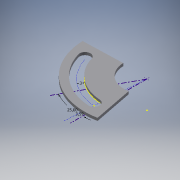
# Autodesk Inventor part: Fixação Painel
Saved by Autodesk Inventor 2019 (Build 230136000, 136)
## iProperties
Created: 2020-05-30
Part Number: Fixação Painel
Material: Generic
Document SubType Name: Modeling
Designer: luiza
Density: 1 g/cm^3
Appearance: Default
Author: luiza
Autodesk Inventor part; units mm, degrees
ref_plane "YZ Plane" through (0, 0, 0) normal (1, 0, 0) x (0, 1, 0)
ref_plane "XZ Plane" through (0, 0, 0) normal (0, 1, 0) x (-1, 0, 0)
ref_plane "XY Plane" through (0, 0, 0) normal (0, 0, 1) x (1, 0, 0)
sketch "Sketch1" plane through (0, 0, 0) normal (0, 1, 0) x (-1, 0, 0)
  line L0 (-630.0209, 427.8421) -> (74.3603, 43.9414)
  line L1 (15.297, -15.1219) -> (53.6419, 55.2333) construction
  line L2 (16.0925, -2.4468) -> (17.9301, 26.8331) construction
  line L3 (27.4797, -11.5343) -> (48.5837, -5.3195) construction
  arc A0 (27.9909, -14.7294) -> (12.8636, -2.6572) centre (15.297, -15.1219) ccw
  circle A1 centre (15.297, -15.1219) radius 27.7 construction
  arc A2 (49.9804, -14.0495) -> (8.6482, 18.9352) centre (15.297, -15.1219) ccw
  arc A3 (38.991, -8.1444) -> (44.7466, -6.4495) centre (41.8688, -7.2969) ccw
  arc A4 (17.2199, 15.5179) -> (16.8441, 9.5296) centre (17.032, 12.5237) ccw
  line L4 (27.9909, -14.7294) -> (49.9804, -14.0495)
  line L5 (12.8636, -2.6572) -> (8.6482, 18.9352)
  arc A5 (44.7466, -6.4495) -> (17.2199, 15.5179) centre (15.297, -15.1219) ccw
  arc A6 (38.991, -8.1444) -> (16.8441, 9.5296) centre (15.297, -15.1219) ccw
  line L6 (15.297, -15.1219) -> (15.297, 30.9021) construction
  line L7 (15.297, -15.1219) -> (61.3209, -15.1219) construction
  point P0 (0, 0)
  dimension "d25" = 45
  dimension "d26" = 25
  dimension "d27" = 25.4
  dimension "d32" = 90
  constraints: 19 point on circle, 16 end point, 7 centre point, 7 point on line, 2 perpendicular, 1 coincident, 1 horizontal, 4 other
  measures "d25" angle of L3 L1
  measures "d26" angle of L2 L1
  measures "d27" diameter of A0
  measures "d32" angle of L7 L6
extrude "Extrusion1" add sketch "Sketch1" along normal blind 1.5
sketch "Sketch2" plane through (0, 0, 0) normal (0, -1, 0) x (1, 0, 0)
  line L0 (-15.297, -15.1219) -> (-49.2057, 27.3648)
  line L1 (-8.6482, 18.9352) -> (-12.8636, -2.6572) projected
  arc A0 (-17.2199, 15.5179) -> (-44.7466, -6.4495) centre (-15.297, -15.1219) ccw projected
  arc A1 (-16.8441, 9.5296) -> (-38.991, -8.1444) centre (-15.297, -15.1219) ccw projected
  circle A2 centre (-32.576, 6.5282) radius 3 construction
  point P0 (0, 0)
  point P1 (-15.297, -15.1219)
  dimension "d36" = 49.64
  constraints: 2 end point, 1 centre point, 1 other
  measures "d36" angle of L1 L0
body "Solid1"
